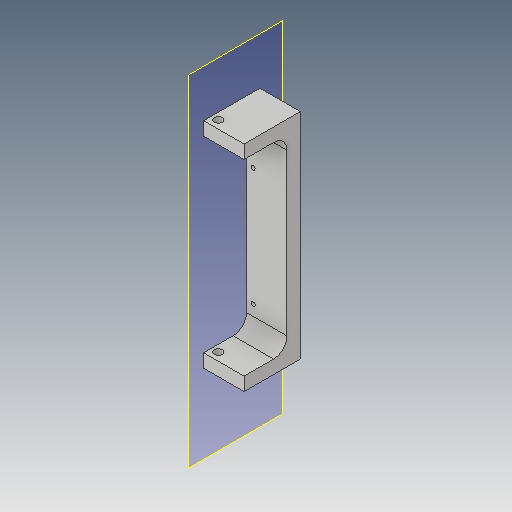
# Autodesk Inventor part: 15_Opentrons_Additional_Slide
Saved by Autodesk Inventor 2019.4 (Build 234330000, 330)
## iProperties
Created: 2021-01-13
Part Number: 15_Opentrons_Additional_Slide
Material: Generic
Document SubType Name: Modeling
Designer: diederichbenedict
Density: 1 g/cm^3
Appearance: Default
Author: diederichbenedict
Autodesk Inventor part; units mm, degrees
ref_plane "YZ Plane" through (0, 0, 0) normal (1, 0, 0) x (0, 1, 0)
ref_plane "XZ Plane" through (0, 0, 0) normal (0, 1, 0) x (-1, 0, 0)
ref_plane "XY Plane" through (0, 0, 0) normal (0, 0, 1) x (1, 0, 0)
ref_plane "Work Plane1" through (-73.1749, 241, 50) normal (-1, 0, 0) x (0, 0, 1)
sketch "Sketch1" plane through (-73.1749, 241, 50) normal (-1, 0, 0) x (0, 0, 1)
  line L0 (-50, -231) -> (-64, -231) projected
  line L1 (-50, -231) -> (-50, -20) projected
  arc A0 (-40, -10) -> (-50, -20) centre (-40, -20) ccw projected
  line L2 (0, -10) -> (-40, -10) projected
  line L3 (0, 0) -> (0, -10) projected
  line L4 (-64, 0) -> (0, 0) projected
  line L5 (-64, 0) -> (-64, -231) projected
  circle A1 centre (-21.5, -69.8271) radius 4 construction
  line L6 (-11, -56.6947) -> (-11, -84.1618) construction
  line L7 (-8, -23.5901) -> (-50, -23.5901)
  line L8 (-50, -23.5901) -> (-50, -33.5901)
  line L9 (-30, -33.5901) -> (-8, -33.5901)
  line L10 (-8, -33.5901) -> (-8, -23.5901)
  line L11 (-50, -183.5901) -> (-8, -183.5901)
  line L12 (-8, -183.5901) -> (-8, -173.5901)
  line L13 (-8, -173.5901) -> (-30, -173.5901)
  line L14 (-50, -173.5901) -> (-50, -183.5901)
  line L15 (-50, -33.5901) -> (-40, -33.5901)
  line L16 (-40, -43.5901) -> (-40, -163.5901)
  line L17 (-40, -173.5901) -> (-50, -173.5901)
  line L18 (-50, -173.5901) -> (-50, -33.5901)
  arc A2 (-30, -33.5901) -> (-40, -43.5901) centre (-30, -43.5901) ccw
  arc A3 (-40, -163.5901) -> (-30, -173.5901) centre (-30, -163.5901) ccw
  point P0 (-50, -241)
  dimension "d0" = 10
  dimension "d1" = 10
  dimension "d2" = 42
  dimension "d3" = 10
  dimension "d4" = 140
  dimension "d5" = 10
  dimension "d18" = 0
  constraints: 24 end point, 7 point on line, 6 parallel, 4 point on circle, 4 tangent, 3 horizontal, 3 perpendicular, 2 centre point, 1 equal radius
  measures "d0" distance of L8.end L7.end
  measures "d1" distance of L12.end L11.end
  measures "d2" distance between parallel lines of L1 L10
  measures "d3" distance of L17.start L17.end
  measures "d4" distance between parallel lines of L13 L15
  measures "d5" radius of A2
  measures "d18" distance between parallel lines of L12 L10
ref_plane "Work Plane2" through (-42.9985, 19.9999, -14.0003) normal (1, 0, 0) x (0, 1, 0)
extrude "Extrusion1" add sketch "Sketch1" against normal up to surface (30.1764 mm away) contours L1 L7 L10 L9 A2 L16 A3 L13 L12 L11
sketch "Sketch2" plane through (-73.1749, 57.4099, 0) normal (0, -1, 0) x (1, 0, 0)
  line L0 (30.1764, 0) -> (30.1764, 42) projected
  line L1 (0, 42) -> (30.1764, 42) projected
  line L2 (0, 0) -> (0, 42) projected
  line L3 (0, 0) -> (30.1764, 0) projected
  circle A0 centre (5, 36) radius 3
  line L4 (0, 42) -> (30.1764, 42) projected
  point P0 (73.1749, 0)
  dimension "d8" = 6
  dimension "d19" = 6
  constraints: 1 centre point
  measures "d8" diameter of A0
  measures "d19" distance from line of A0.centre L4
extrude "Extrusion2" cut sketch "Sketch2" against normal through all contours A0
sketch "Sketch3" plane through (-73.1749, 77.4099, 10) normal (0, 0, 1) x (1, 0, 0)
  arc A0 (7, 91.7198) -> (7, 90.4353) centre (5.7, 91.0776) ccw projected
  circle A1 centre (5, 96.0295) radius 1.4 projected
  circle A2 centre (5, 8.0376) radius 1.4 projected
  point P0 (73.1749, -77.4099)
hole "Hole1" at (-68.1749, 173.4393, 10) at (-68.1749, 85.4474, 10) direction (0, 0, -1) diameter 2.9 end through all both
body "Solid1"
